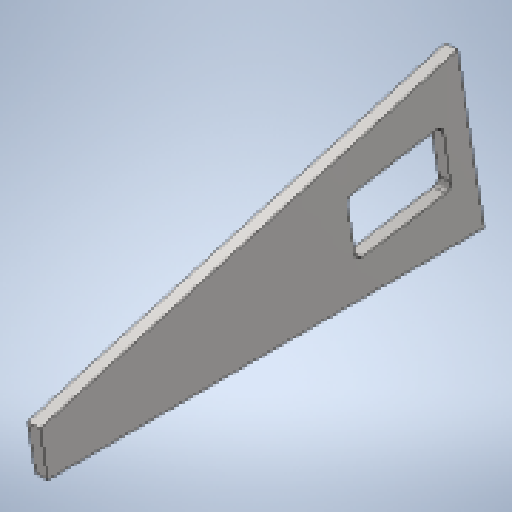
# Autodesk Inventor part: Upright
Saved by Autodesk Inventor 2023.2 (Build 272271000, 271)
## iProperties
Created: 2024-03-17
Part Number: Upright
Material: Stainless Steel
Document SubType Name: Modeling
Designer: Nathan Cai
Mass: 61.8453 g
Surface Area: 60.4703 cm^2
Volume: 7.73066 cm^3
Density: 8 g/cm^3
Appearance: Semi-Polished
Author: Nathan Cai
Autodesk Inventor part; units mm, degrees
ref_plane "YZ Plane" through (0, 0, 0) normal (1, 0, 0) x (0, 1, 0)
ref_plane "XZ Plane" through (0, 0, 0) normal (0, 1, 0) x (-1, 0, 0)
ref_plane "XY Plane" through (0, 0, 0) normal (0, 0, 1) x (1, 0, 0)
sketch "Sketch1" plane through (0, 0, 0) normal (1, 0, 0) x (0, 1, 0)
  line L0 (0, 0) -> (0, 101.6)
  line L1 (0, 0) -> (43.9027, 6.9535)
  line L2 (0, 0) -> (44.45, 0) construction
  line L3 (21.9514, 3.4768) -> (0, 142.0723) construction
  line L4 (9.1448, 33.5942) -> (13.1182, 8.5069)
  line L5 (13.1182, 8.5069) -> (28.7978, 10.9903)
  line L6 (28.7978, 10.9903) -> (24.8244, 36.0776)
  line L7 (24.8244, 36.0776) -> (9.1448, 33.5942)
  line L8 (9.1448, 33.5942) -> (28.7978, 10.9903) construction
  line L9 (13.1182, 8.5069) -> (24.8244, 36.0776) construction
  line L10 (43.9027, 6.9535) -> (12.7, 103.6115)
  line L11 (12.7, 103.6115) -> (0, 101.6)
  circle A0 centre (3.9688, 38.1) radius 1.7526
  arc A1 (6.2444, 44.0282) -> (5.1804, 44.3333) centre (3.9688, 38.1) ccw construction
  arc A2 (7.2299, 46.5956) -> (5.7051, 47.0328) centre (3.9688, 38.1) ccw
  arc A3 (5.2589, 41.4609) -> (4.6557, 41.6339) centre (3.9688, 38.1) ccw
  arc A4 (5.2589, 41.4609) -> (7.2299, 46.5956) centre (6.2444, 44.0282) ccw
  arc A5 (5.7051, 47.0328) -> (4.6557, 41.6339) centre (5.1804, 44.3333) ccw
  line L12 (3.9688, 38.1) -> (6.2444, 44.0282) construction
  line L13 (3.9688, 38.1) -> (10.3188, 38.1) construction
  line L14 (3.9688, 38.1) -> (5.1804, 44.3333) construction
  point P0 (18.9713, 22.2922)
  dimension "d0" = 101.6
  dimension "d1" = 44.45
  dimension "d2" = 9
  dimension "d3" = 25.4
  dimension "d4" = 15.875
  dimension "d6" = 6.35
  dimension "d11" = 12.7
  dimension "d12" = 3.5052
  dimension "d13" = 3.9688
  dimension "d14" = 38.1
  dimension "d15" = 6.35
  dimension "d16" = 69
  dimension "d17" = 10
  dimension "d18" = 5.5
  constraints: 30 end point, 10 point on circle, 6 centre point, 4 parallel, 4 tangent, 3 midpoint, 2 equal length, 2 horizontal, 2 perpendicular, 2 point on line, 1 coincident, 1 vertical
  measures "d0" distance of L0.start L0.end
  measures "d1" distance of L0.start L1.end
  measures "d2" angle of L2 L1
  measures "d3" distance between parallel lines of L5 L7
  measures "d4" distance between parallel lines of L4 L6
  measures "d6" distance between parallel lines of L1 L5
  measures "d11" horizontal distance of L0.end L10.end
  measures "d12" diameter of A0
  measures "d13" distance from line of L0 A0.centre
  measures "d14" distance from line of L2 A0.centre
  measures "d15" radius of A1
  measures "d16" angle of L13 L12
  measures "d17" angle of L12 L14
  measures "d18" diameter of A5
extrude "Extrusion1" add sketch "Sketch1" along normal blind 3.175
fillet "Fillet1" radius 1.5875 4 edges at (1.5875, 24.8244, 36.0776) (1.5875, 9.1448, 33.5942) (1.5875, 13.1182, 8.5069) (1.5875, 28.7978, 10.9903)
body "Solid1"
